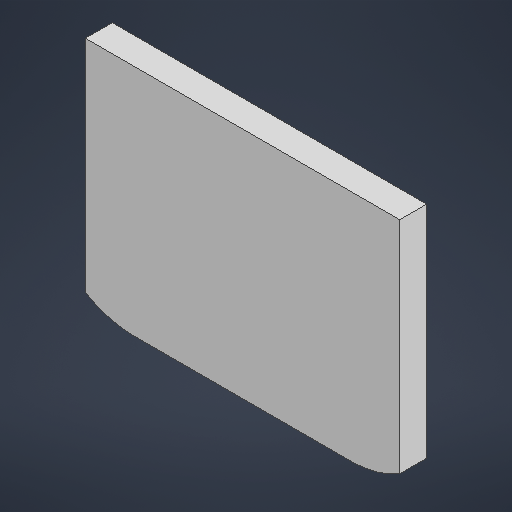
# Autodesk Inventor part: 键盘
Saved by Autodesk Inventor 2025 (Build 290162000, 162)
## iProperties
Created: 2025-11-30
Part Number: 键盘
Material: 常规
Document SubType Name: Modeling
Designer: XH
Density: 1 g/cm^3
Appearance: 默认
Author: XH
Autodesk Inventor part; units mm, degrees
ref_plane "YZ Plane" through (0, 0, 0) normal (1, 0, 0) x (0, 1, 0)
ref_plane "XZ Plane" through (0, 0, 0) normal (0, 1, 0) x (-1, 0, 0)
ref_plane "XY Plane" through (0, 0, 0) normal (0, 0, 1) x (1, 0, 0)
sketch "草图1" plane through (0, 0, 0) normal (0, 0, 1) x (1, 0, 0)
  line L0 (35, -26) -> (-35, -26)
  line L1 (-35, -26) -> (-35, 26)
  line L2 (-35, 26) -> (35, 26)
  line L3 (35, 26) -> (35, -26)
  line L4 (35, -26) -> (-35, 26) construction
  line L5 (-35, -26) -> (35, 26) construction
  point P0 (0, 0)
  dimension "d0" = 70
  dimension "d1" = 52
  constraints: 12 end point, 2 midpoint, 2 parallel, 1 horizontal, 1 perpendicular
  measures "d0" distance of L1.end L2.end
  measures "d1" distance of L0.end L1.end
extrude "拉伸1" add sketch "草图1" along normal blind 6
sketch "草图2" plane through (0, 0, 6) normal (0, 0, 1) x (1, 0, 0)
  line L0 (35, 26) -> (-35, 26) projected
  line L1 (-35, 26) -> (-35, -26) projected
  line L2 (-35, -26) -> (35, -26) projected
  line L3 (35, -26) -> (35, 26) projected
  arc A0 (-35, -23) -> (-25, -26) centre (-23.9099, -4.1996) ccw
  point P0 (0, 0)
  dimension "d4" = 3
  dimension "d5" = 10
  constraints: 2 point on circle, 2 point on line, 1 centre point
  measures "d4" distance from line of L2 A0.start
  measures "d5" distance from line of L1 A0.end
extrude "拉伸2" cut sketch "草图2" against normal blind 6 contours A0 L2 L1
mirror "镜像1" about plane through (0, 0, 0) normal (1, 0, 0) of "拉伸2"
ref_plane "工作平面1" through (0, 0, 0) normal (1, 0, 0) x (0, 1, 0)
